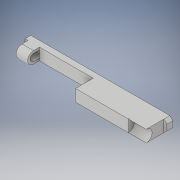
# Autodesk Inventor part: Lolipop
Saved by Autodesk Inventor 2018 (Build 220112000, 112)
## iProperties
Created: 2019-06-07
Part Number: Lolipop
Material: Generic
Document SubType Name: Modeling
Designer: russd
Density: 1 g/cm^3
Appearance: Default
Author: russd
Autodesk Inventor part; units mm, degrees
ref_plane "YZ Plane" through (0, 0, 0) normal (1, 0, 0) x (0, 1, 0)
ref_plane "XZ Plane" through (0, 0, 0) normal (0, 1, 0) x (-1, 0, 0)
ref_plane "XY Plane" through (0, 0, 0) normal (0, 0, 1) x (1, 0, 0)
sketch "Sketch1" plane through (0, 0, 0) normal (0, 0, 1) x (1, 0, 0)
  line L0 (0, 0) -> (152.4, 0)
  line L1 (152.4, 0) -> (152.4, 12.7)
  line L2 (152.4, 12.7) -> (0, 12.7)
  line L3 (0, 12.7) -> (0, 0)
  dimension "d0" = 152.4
  dimension "d1" = 12.7
  constraints: 8 end point, 2 parallel, 1 horizontal, 1 perpendicular
  measures "d0" distance of L2.end L1.end
  measures "d1" distance of L1.end L0.end
sketch "Sketch1 outline for Extrusion1" plane through (0, 0, 0) normal (0, 0, 1) x (1, 0, 0)
  line L0 (0, 12.7) -> (0, 0)
  line L1 (152.4, 12.7) -> (0, 12.7)
  line L2 (152.4, 0) -> (152.4, 12.7)
  line L3 (0, 0) -> (152.4, 0)
extrude "Extrusion1" add sketch "Sketch1 outline for Extrusion1" along normal blind 6.35
chamfer "Chamfer1" distance 3.175 angle 45 2 edges at (152.4, 12.7, 3.175) (152.4, 0, 3.175)
sketch "Sketch2" plane through (0, 0, 6.35) normal (0, 0, 1) x (1, 0, 0)
  line L0 (0, 0) -> (149.225, 0)
  line L1 (149.225, 12.7) -> (0, 12.7)
  line L2 (15.570231, 0) -> (3.175, 0)
  line L3 (3.175, 0) -> (3.175, 12.7)
  line L4 (3.175, 12.7) -> (15.570231, 12.7)
  line L5 (15.570231, 12.7) -> (15.570231, 0)
  point P0 (3.175, 0)
  constraints: 8 end point, 2 parallel, 1 horizontal, 1 perpendicular, 1 point on line
sketch "Sketch2 outline for Extrusion2" plane through (0, 0, 6.35) normal (0, 0, 1) x (1, 0, 0)
  line L0 (15.570231, 0) -> (3.175, 0)
  line L1 (3.175, 0) -> (3.175, 12.7)
  line L2 (3.175, 12.7) -> (15.570231, 12.7)
  line L3 (15.570231, 12.7) -> (15.570231, 0)
extrude "Extrusion2" add sketch "Sketch2 outline for Extrusion2" along normal blind 12.7
fillet "Fillet1" radius 6.35 2 edges at (9.3726, 12.7, 19.05) (9.3726, 0, 19.05)
shell "Shell1" thickness 2.54 removed faces 1 at (15.570231, 8.466667, 10.5834)
sketch "Sketch3" plane through (0, 0, 6.35) normal (0, 0, 1) x (1, 0, 0)
  line L0 (0, 0) -> (149.225, 0)
  line L1 (149.225, 12.7) -> (0, 12.7)
  line L2 (149.225, 0) -> (73.440725, 0)
  line L3 (73.440725, 0) -> (73.440725, 12.7)
  line L4 (73.440725, 12.7) -> (149.225, 12.7)
  line L5 (149.225, 12.7) -> (149.225, 0)
  constraints: 8 end point, 2 parallel, 1 horizontal, 1 perpendicular, 1 point on line
sketch "Sketch3 outline for Extrusion3" plane through (0, 0, 6.35) normal (0, 0, 1) x (1, 0, 0)
  line L0 (149.225, 0) -> (73.440725, 0)
  line L1 (73.440725, 0) -> (73.440725, 12.7)
  line L2 (73.440725, 12.7) -> (149.225, 12.7)
  line L3 (149.225, 12.7) -> (149.225, 0)
extrude "Extrusion3" add sketch "Sketch3 outline for Extrusion3" along normal blind 19.05
sketch "Sketch4" plane through (149.225, 0, 6.35) normal (1, 0, 0) x (0, 0, -1)
  line L0 (-19.05, 12.7) -> (-19.05, 0) projected
  circle A0 centre (-19.05, 6.35) radius 6.35
  point P0 (6.35, 0)
  constraints: 1 midpoint, 1 vertical alignment, 2 other
sketch "Sketch4 outline for Extrusion4" plane through (149.225, 0, 6.35) normal (1, 0, 0) x (0, 0, -1)
  circle A0 centre (-19.05, 6.35) radius 6.35
extrude "Extrusion4" cut sketch "Sketch4 outline for Extrusion4" against normal blind 19.05
body "Solid1"
